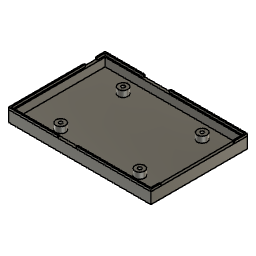
CaseBottom (Autodesk Fusion 360 design; units mm, degrees)
Autodesk Fusion 360 part; units mm, degrees
sketch "Sketch1" plane through (0, 0, 0) normal (0, 0, 1) x (1, 0, 0)
  line L0 (0, 0) -> (102.5, 0)
  line L1 (102.5, 0) -> (102.5, 69.5)
  line L2 (102.5, 69.5) -> (0, 69.5)
  line L3 (0, 69.5) -> (0, 0)
  dimension "d1" = 69.5
  dimension "d2" = 102.5
  constraint horizontal L0
  constraint vertical L1
  constraint horizontal L2
  constraint vertical L3
  constraint coincident L0.start L3.end
  measures "d1" distance of L0 L2
  measures "d2" distance of L1 L3
extrude "Extrude1" add sketch "Sketch1" along normal blind 8 makes body 1
shell "Shell1" thickness 2 removed faces 1 at (34.1667, 46.3333, 8) on bodies 1
sketch "Sketch2" plane through (0, 0, 2) normal (0, 0, 1) x (-1, 0, 0)
  line L0 (-2, -67.5) -> (-2, -2)
  line L1 (-2, -2) -> (-100.5, -2)
  line L2 (-100.5, -2) -> (-100.5, -67.5)
  line L3 (-100.5, -67.5) -> (-2, -67.5)
  circle A0 centre (-82.25, -57.25) radius 3.5
  dimension "d6" = 7
  dimension "d7" = 18.25
  dimension "d8" = 10.25
  measures "d6" diameter of A0
  measures "d7" distance of L2 A0.centre
  measures "d8" distance of L3 A0.centre
extrude "Extrude2" add sketch "Sketch2" along normal blind 4.4 contours A0 bodies 1
sketch "Sketch4" plane through (0, 0, 0) normal (0, 0, -1) x (1, 0, 0)
  line L0 (0, 0) -> (0, -69.5)
  line L1 (0, -69.5) -> (102.5, -69.5)
  line L2 (102.5, -69.5) -> (102.5, 0)
  line L3 (102.5, 0) -> (0, 0)
  circle A0 centre (82.25, -57.25) radius 2.5
  dimension "d11" = 20.25
  dimension "d12" = 12.25
  dimension "d13" = 5
  measures "d11" distance of L2 A0.centre
  measures "d12" distance of L1 A0.centre
  measures "d13" diameter of A0
extrude "Extrude3" cut sketch "Sketch4" against normal blind 3 contours A0 bodies 1
sketch "Sketch5" plane through (0, 0, 6.4) normal (0, 0, 1) x (-1, 0, 0)
  circle A0 centre (-82.25, -57.25) radius 3.5
  circle A1 centre (-82.25, -57.25) radius 1.25
  dimension "d16" = 2.5
  constraint concentric A0 A1
  measures "d16" diameter of A1
extrude "Extrude4" cut sketch "Sketch5" against normal blind 6 contours A1 bodies 1
pattern_linear "R-Pattern1" count 2 spacing 57 along (-1, 0, 0) count 2 spacing 45 along (0, -1, 0) of "Extrude2", "Extrude3", "Extrude4"
sketch "Sketch7" plane through (0, 0, 8) normal (0, 0, 1) x (-1, 0, 0)
  line L0 (-2, -67.5) -> (-100.5, -67.5)
  line L1 (-100.5, -67.5) -> (-100.5, -2)
  line L2 (-100.5, -2) -> (-2, -2)
  line L3 (-2, -2) -> (-2, -67.5)
  line L4 (0, -69.5) -> (0, 0)
  line L5 (0, 0) -> (-102.5, 0)
  line L6 (-102.5, 0) -> (-102.5, -69.5)
  line L7 (-102.5, -69.5) -> (0, -69.5)
  line L8 (0, -69.5) -> (-102.5, -69.5)
  line L9 (-102.5, -69.5) -> (-102.5, 0)
  line L10 (-102.5, 0) -> (0, 0)
  line L11 (0, 0) -> (0, -69.5)
  constraint horizontal L8
  constraint vertical L9
  constraint horizontal L10
  constraint vertical L11
  constraint coincident L5.end L6.start
  constraint coincident L4.start L7.end
extrude "Extrude6" add sketch "Sketch7" along normal blind 1.6 separate body makes body 2
move_face "OffsetFaces1" offset -1 4 faces at (34.8333, 67.5, 8.5333) (2, 45.6667, 8.5333) (67.6667, 2, 8.5333) (100.5, 23.8333, 8.5333) on bodies 2
sketch "Sketch10" plane through (0, 0, 0) normal (-1, 0, 0) x (0, -1, 0)
  line L0 (-69.5, 8) -> (0, 8)
  line L1 (0, 8) -> (0, 9.6)
  line L2 (0, 9.6) -> (-69.5, 9.6)
  line L3 (-69.5, 9.6) -> (-69.5, 8)
  line L4 (-62.75, 9.6) -> (-54.25, 9.6)
  line L5 (-54.25, 9.6) -> (-54.25, 8)
  line L6 (-54.25, 8) -> (-62.75, 8)
  line L7 (-62.75, 8) -> (-62.75, 9.6)
  dimension "d38" = 6.75
  dimension "d39" = 8.5
  constraint horizontal L4
  constraint vertical L5
  constraint horizontal L6
  constraint vertical L7
  constraint coincident L0 L5.end
  constraint coincident L2 L4.start
  measures "d38" distance of L3 L7
  measures "d39" distance of L5 L7
extrude "Extrude10" cut sketch "Sketch10" against normal blind 2 contours L0 L2 L4 L5 L6 L7 bodies 2
sketch "Sketch11" plane through (0, 0, 0) normal (0, -1, 0) x (1, 0, 0)
  line L0 (0, 8) -> (102.5, 8)
  line L1 (102.5, 8) -> (102.5, 9.6)
  line L2 (102.5, 9.6) -> (0, 9.6)
  line L3 (0, 9.6) -> (0, 8)
  line L4 (35.25, 9.6) -> (48.75, 9.6)
  line L5 (48.75, 9.6) -> (48.75, 8)
  line L6 (48.75, 8) -> (35.25, 8)
  line L7 (35.25, 8) -> (35.25, 9.6)
  dimension "d42" = 35.25
  dimension "d43" = 13.5
  constraint horizontal L4
  constraint vertical L5
  constraint horizontal L6
  constraint vertical L7
  constraint coincident L0 L5.end
  constraint coincident L2 L4.start
  measures "d42" distance of L3 L7
  measures "d43" distance of L5 L7
extrude "Extrude11" cut sketch "Sketch11" against normal blind 2 contours L0 L2 L4 L5 L6 L7 bodies 2 makes body 3 at (0.3333, 18.4167, 8)
sketch "Sketch12" plane through (102.5, 0, 0) normal (1, 0, 0) x (0, 1, 0)
  line L0 (0, 8) -> (69.5, 8)
  line L1 (69.5, 8) -> (69.5, 9.6)
  line L2 (69.5, 9.6) -> (0, 9.6)
  line L3 (0, 9.6) -> (0, 8)
  line L4 (7.25, 9.6) -> (60.25, 9.6)
  line L5 (60.25, 9.6) -> (60.25, 8)
  line L6 (60.25, 8) -> (7.25, 8)
  line L7 (7.25, 8) -> (7.25, 9.6)
  dimension "d46" = 7.25
  dimension "d47" = 9.25
  constraint horizontal L4
  constraint vertical L5
  constraint horizontal L6
  constraint vertical L7
  constraint coincident L0 L5.end
  constraint coincident L2 L4.start
  measures "d46" distance of L3 L7
  measures "d47" distance of L1 L5
extrude "Extrude12" cut sketch "Sketch12" against normal blind 2 contours L0 L2 L4 L5 L6 L7 bodies 2 makes body 4 at (84.5833, 0, 9.0667)
sketch "Sketch13" plane through (0, 69.5, 0) normal (0, 1, 0) x (-1, 0, 0)
  line L0 (-102.5, 8) -> (0, 8)
  line L1 (0, 8) -> (0, 9.6)
  line L2 (0, 9.6) -> (-102.5, 9.6)
  line L3 (-102.5, 9.6) -> (-102.5, 8)
  line L4 (-47.25, 9.6) -> (-28.75, 9.6)
  line L5 (-28.75, 9.6) -> (-28.75, 8)
  line L6 (-28.75, 8) -> (-47.25, 8)
  line L7 (-47.25, 8) -> (-47.25, 9.6)
  dimension "d50" = 28.75
  dimension "d51" = 47.25
  constraint horizontal L4
  constraint vertical L5
  constraint horizontal L6
  constraint vertical L7
  constraint coincident L0 L5.end
  constraint coincident L2 L4.start
  measures "d50" distance of L1 L5
  measures "d51" distance of L1 L7
extrude "Extrude13" cut sketch "Sketch13" against normal blind 2 contours L0 L2 L4 L5 L6 L7 bodies 2 makes body 5 at (19.1667, 69.5, 9.0667)
equation "d38 = 4.5 mm + 2.25 mm"
equation "d42 = 33 mm + 2.25 mm"
equation "d46 = 5 mm + 2.25 mm"
equation "d47 = 7 mm + 2.25 mm"
equation "d50 = 26.5 mm + 2.25 mm"
equation "d51 = 45 mm + 2.25 mm"
